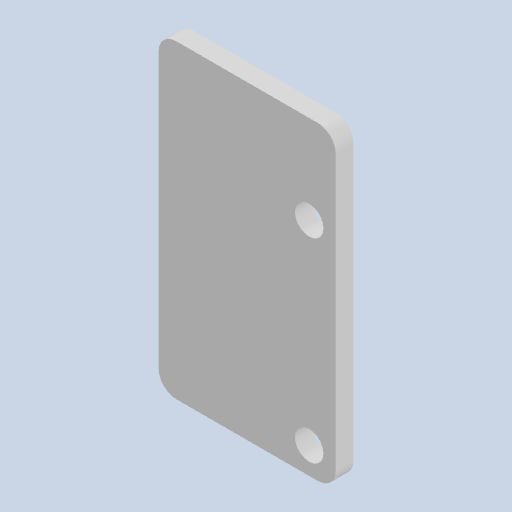
# Autodesk Inventor part: comutation_motorboard
Saved by Autodesk Inventor 2022 (Build 260153000, 153)
## iProperties
Created: 2024-11-26
Part Number: comutation_motorboard
Material: Типовые
Document SubType Name: Modeling
Designer: Andrey
Density: 1 g/cm^3
Appearance: По умолчанию
Author: Andrey
Autodesk Inventor part; units mm, degrees
ref_plane "YZ Plane" through (0, 0, 0) normal (1, 0, 0) x (0, 1, 0)
ref_plane "XZ Plane" through (0, 0, 0) normal (0, 1, 0) x (-1, 0, 0)
ref_plane "XY Plane" through (0, 0, 0) normal (0, 0, 1) x (1, 0, 0)
sketch "Эскиз1" plane through (0, 0, 0) normal (0, 0, 1) x (1, 0, 0)
  line L0 (10, -17.5) -> (-10, -17.5)
  line L1 (-10, -17.5) -> (-10, 17.5)
  line L2 (-10, 17.5) -> (10, 17.5)
  line L3 (10, 17.5) -> (10, -17.5)
  line L4 (10, -17.5) -> (-10, 17.5) construction
  line L5 (-10, -17.5) -> (10, 17.5) construction
  point P0 (0, 0)
  dimension "d0" = 20
  dimension "d1" = 35
  constraints: 12 end point, 2 midpoint, 2 parallel, 1 horizontal, 1 perpendicular
  measures "d0" distance of L1.end L2.end
  measures "d1" distance of L0.end L1.end
extrude "Выдавливание1" add sketch "Эскиз1" along normal blind 2
fillet "Сопряжение1" radius 2 4 edges at (-10, 17.5, 1) (10, 17.5, 1) (10, -17.5, 1) (-10, -17.5, 1)
sketch "Эскиз2" plane through (0, 0, 0) normal (0, 0, -1) x (-1, 0, 0)
  circle A0 centre (-7, 7.5) radius 2.1 projected
  circle A1 centre (-7, -14.5) radius 2.1 projected
  line L0 (-5.7982, 10.5) -> (-5.7982, 18.5) projected
  line L1 (-5.7982, 18.5) -> (-8, 18.5) projected
  arc A2 (-8, 18.5) -> (-11, 15.5) centre (-8, 15.5) ccw projected
  line L2 (-11, 15.5) -> (-11, 2.5) projected
  arc A3 (-11, -15.5) -> (-8, -18.5) centre (-8, -15.5) ccw projected
  line L3 (-8, -18.5) -> (8, -18.5) projected
  arc A4 (8, -18.5) -> (11, -15.5) centre (8, -15.5) ccw projected
  line L4 (11, 6) -> (11, 10.5) projected
  line L5 (11, 10.5) -> (-5.7982, 10.5) projected
  circle A5 centre (-7, -14.5) radius 1.6
  circle A6 centre (-7, 7.5) radius 1.6
  line L6 (-11, 2.5) -> (-4, 2.5) projected
  line L7 (-4, 2.5) -> (-4, -9.5) projected
  line L8 (-4, -9.5) -> (-11, -9.5) projected
  line L9 (11, -6) -> (4, -6) projected
  line L10 (4, -6) -> (4, 6) projected
  line L11 (4, 6) -> (11, 6) projected
  line L12 (-11, -9.5) -> (-11, -15.5) projected
  line L13 (11, -15.5) -> (11, -6) projected
  point P0 (0, 0)
  dimension "d5" = 3.2
  dimension "d6" = 3.2
  constraints: 2 centre point, 2 coincident
  measures "d5" diameter of A5
  measures "d6" diameter of A6
extrude "Выдавливание2" cut sketch "Эскиз2" against normal blind 2 contours A5 | A6
